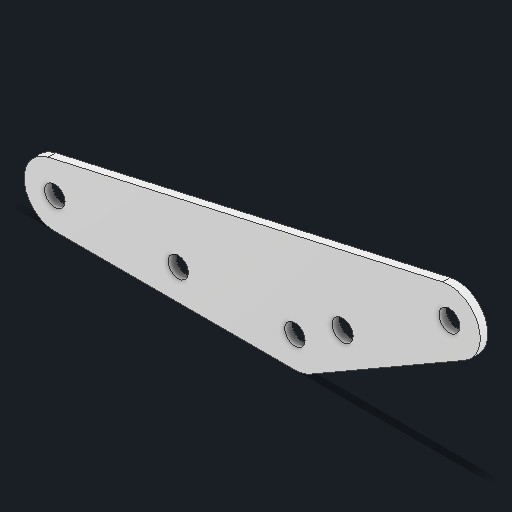
# Autodesk Inventor part: 60 Degree Gusset
Saved by Autodesk Inventor 2025.1 (Build 291241000, 241)
## iProperties
Created: 2024-10-22
Part Number: 60 Degree Gusset
Material: Acetal Resin, White
Document SubType Name: Sheet Metal
Designer: averey
Density: 1.425 g/cm^3
Appearance: Smooth - White
Mass: 2.47081 g
Surface Area: 25.8634 cm^2
Volume: 1.7339 cm^3
Flat Pattern Width: 2.35976 cm
Flat Pattern Length: 9.59773 cm
Flat Pattern Area: 22.6483 cm^2
Sheet Metal Rule: Default_mm
Sheet Metal Width: 0.929 in
Sheet Metal Length: 3.779 in
Sheet Metal Area: 3.510 in^2
Author: averey
Autodesk Inventor part; units mm, degrees
ref_plane "YZ Plane" through (0, 0, 0) normal (1, 0, 0) x (0, 1, 0)
ref_plane "XZ Plane" through (0, 0, 0) normal (0, 1, 0) x (-1, 0, 0)
ref_plane "XY Plane" through (0, 0, 0) normal (0, 0, 1) x (1, 0, 0)
sketch "main" plane through (0, 0, 0) normal (0, 0, 1) x (1, 0, 0)
  circle A0 centre (15.0202, -6.3416) radius 2.1844
  circle A1 centre (37.0172, 6.3584) radius 2.1844
  arc A2 (40.1922, 0.8591) -> (33.8536, 11.8642) centre (37.0172, 6.3584) ccw
  line L0 (-44.2105, -18.3536) -> (5.2134, -18.3536)
  line L1 (40.1922, 0.8591) -> (8.3884, -17.5028)
  circle A3 centre (5.2134, -12.0036) radius 2.0955
  arc A4 (5.2134, -18.3536) -> (8.3884, -17.5028) centre (5.2134, -12.0036) ccw
  line L2 (5.2134, -12.0036) -> (43.3134, -12.0036) construction
  arc A5 (-45.6106, -5.8098) -> (-44.2105, -18.3536) centre (-44.2105, -12.0036) ccw
  line L3 (33.8536, 11.8642) -> (68.8891, 11.8642) construction
  line L4 (-45.6106, -5.8098) -> (35.6171, 12.5521)
  circle A6 centre (-18.8105, -12.0036) radius 2.0955
  circle A7 centre (-44.2105, -12.0036) radius 2.0955
  point P0 (-0.7926, -1.6009)
  dimension "d3" = 12.7
  dimension "d7" = 4.191
  dimension "d8" = 6.35
  dimension "d13" = 25.4
  dimension "d16" = 4.191
  measures "d3" diameter of A2
  measures "d7" diameter of A3
  measures "d8" radius of A4
  measures "d13" distance of A1.centre A0.centre
  measures "d16" diameter of A7
sketch "Sketch1" plane through (0, 0, 0) normal (0, 0, 1) x (1, 0, 0)
  circle A0 centre (46.5307, 5.662) radius 2.1844
  circle A1 centre (68.5277, 18.362) radius 2.1844
  arc A2 (71.7027, 12.8627) -> (65.3641, 23.8678) centre (68.5277, 18.362) ccw
  line L0 (-12.7, -6.35) -> (36.7239, -6.35)
  line L1 (71.7027, 12.8627) -> (39.8989, -5.4993)
  circle A3 centre (36.7239, 0) radius 2.0955
  arc A4 (36.7239, -6.35) -> (39.8989, -5.4993) centre (36.7239, 0) ccw
  line L2 (36.7239, 0) -> (74.8239, 0) construction
  arc A5 (-14.1001, 6.1937) -> (-12.7, -6.35) centre (-12.7, 0) ccw
  line L3 (65.3641, 23.8678) -> (100.3996, 23.8678) construction
  line L4 (-14.1001, 6.1937) -> (67.1276, 24.5557)
  circle A6 centre (12.7, 0) radius 2.0955
  circle A7 centre (-12.7, 0) radius 2.0955
  point P0 (0, 0)
extrude "Extrusion1" add sketch "Sketch1" along normal blind 1.5875
equation "\"BendRadius\" = Thickness"
equation "\"BendReliefWidth\" = Thickness"
equation "\"BendReliefDepth\" = 0.5 * Thickness"
equation "\"CornerReliefSize\" = 4 * Thickness"
equation "\"MinimumRemnant\" = 2 * Thickness"
equation "\"TransitionRadius\" = BendRadius"
equation "\"JacobiRadiusSize\" = BendRadius"
equation "\"GapSize\" = Thickness"
equation "\"Thickness\" = 1.5875"
body "Solid1"
